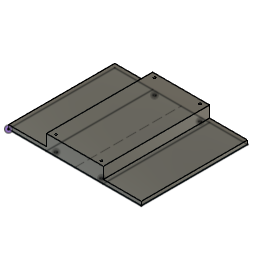
Platform_Riser (Autodesk Fusion 360 design; units mm, degrees)
part number: 2025-10-16-22-08-15-071
Autodesk Fusion 360 part; units mm, degrees
sketch "Sketch1" plane through (0, 0, 0) normal (0, 0, 1) x (1, 0, 0)
  line L0 (0, 0) -> (175, 0)
  line L1 (175, 0) -> (175, 140)
  line L2 (175, 140) -> (0, 140)
  line L3 (0, 140) -> (0, 0)
  line L4 (50, 140) -> (50, 0)
  line L5 (125, 140) -> (125, 0)
  circle A0 centre (57.5, 5) radius 1.35
  circle A1 centre (117.5, 5) radius 1.35
  line L6 (87.5, 0) -> (87.5, 140) construction
  circle A2 centre (57.5, 135) radius 1.35
  circle A3 centre (117.5, 135) radius 1.35
  dimension "d1" = 140
  dimension "d2" = 175
  dimension "d3" = 50
  dimension "d4" = 50
  dimension "d5" = 2.7
  dimension "d6" = 5
  dimension "d7" = 2.7
  dimension "d8" = 5
  dimension "d10" = 60
  dimension "d11" = 2.7
  dimension "d12" = 2.7
  dimension "d13" = 60
  dimension "d14" = 5
  dimension "d15" = 5
  constraint horizontal L0
  constraint vertical L1
  constraint horizontal L2
  constraint vertical L3
  constraint coincident L0.start L3.end
  constraint coincident L2 L4.start
  constraint coincident L0 L4.end
  constraint perpendicular L0 L4
  constraint coincident L2 L5.start
  constraint coincident L0 L5.end
  constraint perpendicular L0 L5
  constraint midpoint L0 L6.start
  constraint midpoint L2 L6.end
  constraint symmetric A0.centre A1.centre L6
  constraint symmetric L6 A2.centre A3.centre
  measures "d1" distance of L0.start L2.end
  measures "d2" distance of L0.start L0.end
  measures "d3" distance of L3 L4
  measures "d4" distance of L1 L5
  measures "d5" diameter of A0
  measures "d6" distance of L0 A0.centre
  measures "d7" diameter of A1
  measures "d8" distance of L0 A1.centre
  measures "d10" distance of A0.centre A1.centre
  measures "d11" diameter of A2
  measures "d12" diameter of A3
  measures "d13" distance of A2.centre A3.centre
  measures "d14" distance of L2 A2.centre
  measures "d15" distance of L2 A3.centre
extrude "Extrude1" add sketch "Sketch1" along normal blind 20 contours L0 L2 L4 L5
extrude "Extrude2" add sketch "Sketch1" along normal blind 15 contours A0 | A1 | A2 | A3
extrude "Extrude3" add sketch "Sketch1" along normal blind 5 contours L0 L2 L3 L4 | L0 L1 L2 L5
